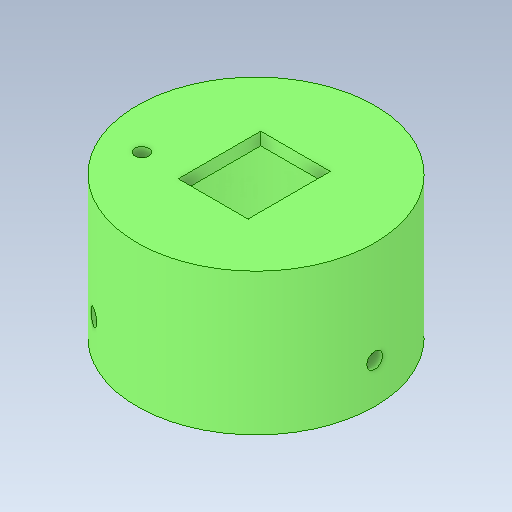
# Autodesk Inventor part: Gauge Housing
Saved by Autodesk Inventor 2020 (Build 240168000, 168)
## iProperties
Created: 2018-03-07
Part Number: Gauge Housing
Material: Generic
Document SubType Name: Modeling
Designer: Alex
Density: 1 g/cm^3
Appearance: Default
Description: 3D Printed Gauge Housing
Vendor: n/a
Author: Alex
Autodesk Inventor part; units mm, degrees
ref_plane "YZ Plane" through (0, 0, 0) normal (1, 0, 0) x (0, 1, 0)
ref_plane "XZ Plane" through (0, 0, 0) normal (0, 1, 0) x (-1, 0, 0)
ref_plane "XY Plane" through (0, 0, 0) normal (0, 0, 1) x (1, 0, 0)
sketch "Sketch1" plane through (0, 0, 0) normal (0, 0, 1) x (1, 0, 0)
  line L0 (21.2725, 0) -> (23.8125, 0)
  line L1 (23.8125, 0) -> (23.8125, 28.3972)
  line L2 (23.8125, 28.3972) -> (6.985, 28.3972)
  line L3 (21.2725, 25.8572) -> (21.2725, 0)
  line L4 (0, -5.6794) -> (0, 34.0766) projected
  line L5 (6.985, 25.8572) -> (6.985, 28.3972)
  line L6 (6.985, 25.8572) -> (21.2725, 25.8572)
  point P0 (0, 0)
  dimension "d5" = 28.3972
  dimension "d10" = 21.2725
  dimension "d13" = 2.54
  dimension "d22" = 6.985
  dimension "d50" = 2.54
  constraints: 12 end point, 2 horizontal, 2 perpendicular, 1 horizontal alignment, 1 vertical
  measures "d5" distance between parallel lines of L0 L2
  measures "d10" distance from line of point (0, 0) L3
  measures "d13" distance between parallel lines of L3 L1
  measures "d22" distance from line of L2.end L4
  measures "d50" distance of L5.start L2.end
revolve "Revolution1" add sketch "Sketch1" angle 360 about axis through (0, -10, 0) along (0, 1, 0)
sketch "Sketch4" plane through (0, 0, 0) normal (1, 0, 0) x (0, 1, 0)
  circle A0 centre (8.001, 0) radius 1.5875
  point P0 (0, 0)
  dimension "d33" = 3.175
  dimension "d34" = 8.001
  constraints: 1 centre point, 1 horizontal alignment
  measures "d33" diameter of A0
  measures "d34" distance of A0.centre point (0, 0)
extrude "Extrusion2" cut sketch "Sketch4" along normal through all
pattern_circular "Circular Pattern1" count 3 over 360 about axis through (0, 14.1986, 0) along (0, -1, 0) of "Extrusion2"
sketch "Sketch5" plane through (0, 28.3972, 0) normal (0, 1, 0) x (1, 0, 0)
  line L0 (6.985, 7.9248) -> (-6.985, 7.9248)
  line L1 (-6.985, 7.9248) -> (-6.985, -8.5852)
  line L2 (-6.985, -8.5852) -> (6.985, -8.5852)
  line L3 (6.985, -8.5852) -> (6.985, 7.9248)
  line L4 (6.985, 7.9248) -> (-6.985, -8.5852) construction
  line L5 (-6.985, 7.9248) -> (6.985, -8.5852) construction
  circle A0 centre (0, 0) radius 6.985 construction
  point P0 (0, -0.3302)
  dimension "d51" = 13.97
  dimension "d52" = 16.51
  dimension "d56" = 0.3302
  constraints: 12 end point, 2 parallel, 1 horizontal, 1 midpoint, 1 perpendicular, 1 vertical alignment
  measures "d51" distance of L2.end L1.end
  measures "d52" distance of L0.end L1.end
  measures "d56" distance of point (0, -0.33) A0.centre
extrude "Extrusion3" cut sketch "Sketch5" against normal through all
sketch "Sketch6" plane through (0, 28.3972, 0) normal (0, 1, 0) x (1, 0, 0)
  circle A0 centre (-15.24, -7.62) radius 1.3959
  line L0 (0, 0) -> (-15.24, -7.62) construction
  line L1 (-15.24, -7.62) -> (0, -7.62) construction
  line L2 (0, -7.62) -> (0, 0) construction
  dimension "d59" = 7.62
  dimension "d60" = 15.24
  constraints: 6 end point, 1 centre point, 1 coincident, 1 perpendicular
  measures "d59" distance of L1.end L0.start
  measures "d60" distance of L0.end L1.end
extrude "Extrusion4" cut sketch "Sketch6" against normal through all
body "Solid1"
